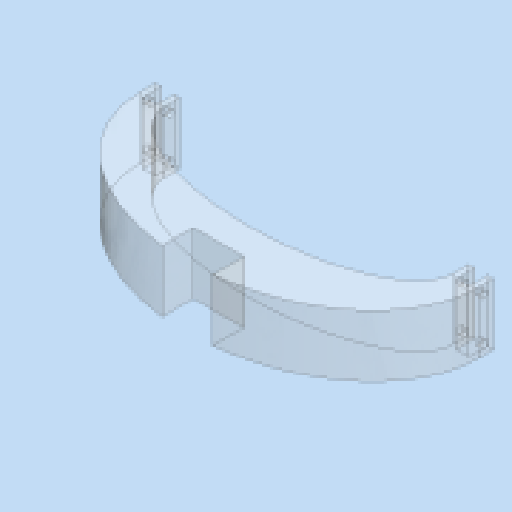
# Autodesk Inventor part: CurvedSeatHolder
Saved by Autodesk Inventor 2023 (Build 270158000, 158)
## iProperties
Created: 2026-03-19
Part Number: CurvedSeatHolder
Material: PET Plastic
Document SubType Name: Modeling
Designer: Nathann
Density: 1.541 g/cm^3
Appearance: Polycarbonate - Clear
Mass: 7081.2 g
Surface Area: 2618.59 cm^2
Volume: 4595.2 cm^3
Author: Nathann
Autodesk Inventor part; units mm, degrees
ref_plane "YZ Plane" through (0, 0, 0) normal (1, 0, 0) x (0, 1, 0)
ref_plane "XZ Plane" through (0, 0, 0) normal (0, 1, 0) x (-1, 0, 0)
ref_plane "XY Plane" through (0, 0, 0) normal (0, 0, 1) x (1, 0, 0)
sketch "Sketch1" plane through (0, 0, 0) normal (0, 1, 0) x (-1, 0, 0)
  line L0 (0, 20.9385) -> (0, -224.0391)
  ellipse E0 centre (275, -2.2065) end of major axis (0, -2.2065) minor radius 200 (275, 197.7935) -> (0, -2.2065) ccw
  ellipse E1 centre (275, -2.2065) end of major axis (40, -2.2065) minor radius 100 (275, 97.7935) -> (40, -2.2065) ccw
  line L1 (0, -2.2065) -> (40, -2.2065)
  line L2 (30.5, -2.2065) -> (9.5, -2.2065)
  line L3 (9.5, -2.2065) -> (9.5, 2.7935)
  line L4 (9.5, 2.7935) -> (30.5, 2.7935)
  line L5 (30.5, 2.7935) -> (30.5, -2.2065)
  line L6 (0, -2.2065) -> (9.5, -2.2065)
  line L7 (9.5, -2.2065) -> (9.5, -27.2065)
  line L8 (9.5, -27.2065) -> (0, -27.2065)
  line L9 (0, -27.2065) -> (0, -2.2065)
  line L10 (30.5, -2.2065) -> (40, -2.2065)
  line L11 (40, -2.2065) -> (40, -27.2065)
  line L12 (40, -27.2065) -> (30.5, -27.2065)
  line L13 (30.5, -27.2065) -> (30.5, -2.2065)
  line L14 (275, -2.2065) -> (275, 197.7935)
  line L15 (550, 20.9385) -> (550, -224.0391)
  ellipse E2 centre (275, -2.2065) end of major axis (550, -2.2065) minor radius 200 (550, -2.2065) -> (275, 197.7935) ccw
  ellipse E3 centre (275, -2.2065) end of major axis (510, -2.2065) minor radius 100 (510, -2.2065) -> (275, 97.7935) ccw
  line L16 (550, -2.2065) -> (510, -2.2065)
  line L17 (519.5, -2.2065) -> (540.5, -2.2065)
  line L18 (540.5, -2.2065) -> (540.5, 2.7935)
  line L19 (540.5, 2.7935) -> (519.5, 2.7935)
  line L20 (519.5, 2.7935) -> (519.5, -2.2065)
  line L21 (550, -2.2065) -> (540.5, -2.2065)
  line L22 (540.5, -2.2065) -> (540.5, -27.2065)
  line L23 (540.5, -27.2065) -> (550, -27.2065)
  line L24 (550, -27.2065) -> (550, -2.2065)
  line L25 (519.5, -2.2065) -> (510, -2.2065)
  line L26 (510, -2.2065) -> (510, -27.2065)
  line L27 (510, -27.2065) -> (519.5, -27.2065)
  line L28 (519.5, -27.2065) -> (519.5, -2.2065)
  point P0 (40, -2.2065)
  point P1 (0, -27.2065)
  dimension "d7" = 275
  dimension "d8" = 235
  dimension "d9" = 100
  dimension "d10" = 200
  dimension "d13" = 21
  dimension "d14" = 9.5
  dimension "d15" = 5
  dimension "d16" = 9.5
  dimension "d17" = 9.5
  dimension "d18" = 25
  dimension "d19" = 25
  dimension "d20" = 30
  constraints: 58 end point, 13 symmetric about line, 7 point on line, 7 vertical, 6 parallel, 4 horizontal, 3 perpendicular, 2 coincident, 1 midpoint, 16 other
  measures "d13" distance of L3.end L4.end
  measures "d14" distance between parallel lines of L0 L3
  measures "d15" distance of L4.end L2.start
  measures "d16" distance of L7.end L8.end
  measures "d17" distance of L11.end L12.end
  measures "d18" distance of L12.end L2.start
  measures "d19" distance of L6.end L7.end
  measures "d20" distance between parallel lines of L12 L4
extrude "Extrusion1" add sketch "Sketch1" along normal blind 100 contours L1 L7 L8 L0 | E0 L14 E1 L1 L5 L4 L3 | E2 L16 L18 L19 L20 E3 L14 | L15 L23 L22 L16 | L1 L11 L12 L13 | L16 L28 L27 L26
sketch "Sketch2" plane through (0, 100, 0) normal (0, 1, 0) x (1, 0, 0)
  line L0 (-234, -145) -> (-316, -145)
  line L1 (-316, -145) -> (-316, -247)
  line L2 (-316, -247) -> (-234, -247)
  line L3 (-234, -247) -> (-234, -145)
  point P0 (0, 0)
  point P1 (-275, -145)
  dimension "d21" = 102
  dimension "d22" = 82
  dimension "d23" = 234
  dimension "d24" = 145
  constraints: 8 end point, 2 parallel, 1 horizontal, 1 midpoint, 1 perpendicular
  measures "d21" distance of L2.end L0.start
  measures "d22" distance of L1.end L2.end
  measures "d23" distance from line of point (0, 0) L3
  measures "d24" vertical distance of point (0, 0) point (-275, -145)
extrude "Extrusion2" cut sketch "Sketch2" against normal blind 300
sketch "Sketch3" plane through (-550, 0, -27.2065) normal (-1, 0, 0) x (0, 0, 1)
  circle A0 centre (15, 15) radius 5.5
  circle A1 centre (15, 85) radius 5.5
  line L0 (0, 0) -> (0, 100) projected
  line L1 (0, 0) -> (25, 0) projected
  line L2 (0, 100) -> (25, 100) projected
  point P0 (27.2065, 0)
  dimension "d27" = 11
  dimension "d28" = 11
  dimension "d29" = 15
  dimension "d30" = 15
  dimension "d31" = 15
  dimension "d32" = 15
  constraints: 2 centre point
  measures "d27" diameter of A0
  measures "d28" diameter of A1
  measures "d29" distance from line of L0 A0.centre
  measures "d30" distance from line of L1 A0.centre
  measures "d31" distance from line of L2 A1.centre
  measures "d32" distance from line of L0 A1.centre
extrude "Extrusion3" cut sketch "Sketch3" against normal blind 700
body "Solid1"
